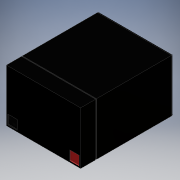
# Autodesk Inventor part: battery
Saved by Autodesk Inventor 2016 (Build 200138000, 138)
## iProperties
Created: 2016-05-30
Part Number: battery
Material: ABS Plastic
Document SubType Name: Modeling
Designer: Henrik Samuelsson
Density: 1.06 g/cm^3
Appearance: Smooth - White
Author: Henrik Samuelsson
Autodesk Inventor part; units mm, degrees
ref_plane "YZ Plane" through (0, 0, 0) normal (1, 0, 0) x (0, 1, 0)
ref_plane "XZ Plane" through (0, 0, 0) normal (0, 1, 0) x (-1, 0, 0)
ref_plane "XY Plane" through (0, 0, 0) normal (0, 0, 1) x (1, 0, 0)
sketch "Sketch1" plane through (0, 0, 0) normal (0, 1, 0) x (-1, 0, 0)
  line L0 (0, 0) -> (79, 0)
  line L1 (79, 0) -> (79, -56)
  line L2 (79, -56) -> (0, -56)
  line L3 (0, -56) -> (0, 0)
  dimension "d0" = 56
  dimension "d1" = 79
  constraints: 8 end point, 2 parallel, 1 horizontal, 1 perpendicular
  measures "d0" distance of L1.end L0.end
  measures "d1" distance of L2.end L1.end
extrude "Extrusion1" add sketch "Sketch1" along normal blind 82
sketch "Sketch4" plane through (0, 0, 0) normal (0, -1, 0) x (1, 0, 0)
  line L0 (-78.5, -0.5) -> (-0.5, -0.5)
  line L1 (-0.5, -0.5) -> (-0.5, -55.5)
  line L2 (-0.5, -55.5) -> (-78.5, -55.5)
  line L3 (-78.5, -55.5) -> (-78.5, -0.5)
  line L4 (-78.5, -0.5) -> (-0.5, -55.5) construction
  line L5 (-0.5, -0.5) -> (-78.5, -55.5) construction
  line L6 (0, 0) -> (-79, 0) projected
  line L7 (-79, 0) -> (-79, -56) projected
  line L8 (-79, -56) -> (0, -56) projected
  line L9 (0, -56) -> (0, 0) projected
  point P0 (-39.5, -28)
  dimension "d4" = 0.5
  dimension "d5" = 0.5
  dimension "d7" = 0.5
  dimension "d8" = 0.5
  constraints: 12 end point, 2 midpoint, 2 parallel, 1 horizontal, 1 perpendicular
  measures "d4" horizontal distance of L6.start L0.end
  measures "d5" distance from line of L8 L1.end
  measures "d7" distance from line of L6 L0.end
  measures "d8" distance from line of L7 L2.end
extrude "Extrusion2" add sketch "Sketch4" along normal blind 1 contours L0 L1 L2 L3
sketch "Sketch5" plane through (0, -1, 0) normal (0, -1, 0) x (1, 0, 0)
  line L0 (-79, 0) -> (0, 0)
  line L1 (0, 0) -> (0, -56)
  line L2 (0, -56) -> (-79, -56)
  line L3 (-79, -56) -> (-79, 0)
  line L4 (-79, 0) -> (0, -56) construction
  line L5 (0, 0) -> (-79, -56) construction
  line L6 (0, -56) -> (0, 0) projected
  line L7 (-79, -56) -> (0, -56) projected
  line L8 (0, 0) -> (-79, 0) projected
  line L9 (-79, 0) -> (-79, -56) projected
  point P0 (-39.5, -28)
  constraints: 12 end point, 4 collinear, 2 midpoint, 2 parallel, 1 horizontal, 1 perpendicular
extrude "Extrusion3" add sketch "Sketch5" along normal blind 16
fillet "Fillet1" radius 2 4 edges at (-39.5, 82, -56) (0, 82, -28) (-39.5, 82, 0) (-79, 82, -28)
sketch "Sketch6" plane through (0, -17, 0) normal (0, -1, 0) x (1, 0, 0)
  line L0 (-11.5, -44.5) -> (-1.5, -44.5)
  line L1 (-1.5, -44.5) -> (-1.5, -54.5)
  line L2 (-1.5, -54.5) -> (-11.5, -54.5)
  line L3 (-11.5, -54.5) -> (-11.5, -44.5)
  line L4 (-11.5, -44.5) -> (-1.5, -54.5) construction
  line L5 (-1.5, -44.5) -> (-11.5, -54.5) construction
  line L6 (0, -56) -> (0, 0) projected
  line L7 (-79, -56) -> (0, -56) projected
  line L8 (-79, 0) -> (-79, -56) projected
  line L9 (-77.5, -44.5) -> (-67.5, -44.5)
  line L10 (-67.5, -44.5) -> (-67.5, -54.5)
  line L11 (-67.5, -54.5) -> (-77.5, -54.5)
  line L12 (-77.5, -54.5) -> (-77.5, -44.5)
  line L13 (-77.5, -44.5) -> (-67.5, -54.5) construction
  line L14 (-67.5, -44.5) -> (-77.5, -54.5) construction
  point P0 (-6.5, -49.5)
  point P1 (-72.5, -49.5)
  dimension "d14" = 10
  dimension "d15" = 10
  dimension "d16" = 1.5
  dimension "d17" = 1.5
  dimension "d18" = 10
  dimension "d19" = 10
  dimension "d20" = 1.5
  dimension "d21" = 1.5
  constraints: 24 end point, 4 midpoint, 4 parallel, 2 horizontal, 2 perpendicular
  measures "d14" distance of L1.end L2.end
  measures "d15" distance of L0.end L1.end
  measures "d16" distance from line of L6 L1.end
  measures "d17" distance between parallel lines of L7 L2
  measures "d18" distance of L10.end L11.end
  measures "d19" distance of L9.end L10.end
  measures "d20" distance between parallel lines of L7 L11
  measures "d21" distance from line of L8 L11.end
extrude "Extrusion4" cut sketch "Sketch6" against normal blind 0.5
fillet "Fillet2" radius 0.5 4 edges at (-72.5, -16.5, -44.5) (-77.5, -16.5, -49.5) (-72.5, -16.5, -54.5) (-67.5, -16.5, -49.5)
fillet "Fillet3" radius 0.5 4 edges at (-11.5, -16.5, -49.5) (-6.5, -16.5, -44.5) (-6.5, -16.5, -54.5) (-1.5, -16.5, -49.5)
body "Solid1"
